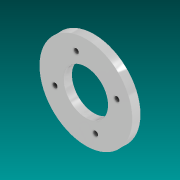
# Autodesk Inventor part: lagerblokje
Saved by Autodesk Inventor 2020.3 (Build 243373000, 373)
## iProperties
Created: 2020-05-22
Part Number: lagerblokje
Material: Aluminum 6061
Document SubType Name: Modeling
Designer: Svend
Density: 2.7 g/cm^3
Appearance: Aluminum - Polished
Author: Svend
Autodesk Inventor part; units mm, degrees
ref_plane "YZ Plane" through (0, 0, 0) normal (1, 0, 0) x (0, 1, 0)
ref_plane "XZ Plane" through (0, 0, 0) normal (0, 1, 0) x (-1, 0, 0)
ref_plane "XY Plane" through (0, 0, 0) normal (0, 0, 1) x (1, 0, 0)
ref_plane "Work Plane1" through (0, 0, 0) normal (0, 0, 1) x (1, 0, 0)
ref_plane "Work Plane2" through (0, 0, 0) normal (0, 0, 1) x (1, 0, 0)
sketch "Sketch2" plane through (0, 0, 0) normal (0, 0, 1) x (1, 0, 0)
  circle A0 centre (-137.1735, 0) radius 1.55
  circle A1 centre (-165.1735, -28) radius 1.55
  circle A2 centre (-165.1735, 28) radius 1.55
  circle A3 centre (-184.9724, -19.799) radius 1.55
  circle A4 centre (-145.3745, 19.799) radius 1.55
  circle A5 centre (-145.3745, -19.799) radius 1.55
  circle A6 centre (-184.9724, 19.799) radius 1.55
  circle A7 centre (-193.1735, 0) radius 1.55
  circle A8 centre (-165.1735, 0) radius 32.5
  circle A9 centre (-165.1735, 0) radius 22.8355
  circle A10 centre (-165.1735, 0) radius 11
  arc A11 (-152.3597, 3.5298) -> (-152.6156, 4.3532) centre (-149.894, 4.7473) ccw
  arc A12 (-152.6156, 4.3532) -> (-168.7032, 12.8137) centre (-165.1735, 0) ccw
  arc A13 (-168.7032, 12.8137) -> (-169.5266, 12.5579) centre (-169.9208, 15.2795) ccw
  arc A14 (-169.5266, 12.5579) -> (-177.9872, -3.5298) centre (-165.1735, 0) ccw
  arc A15 (-177.9872, -3.5298) -> (-177.7313, -4.3532) centre (-180.4529, -4.7473) ccw
  arc A16 (-177.7313, -4.3532) -> (-161.6437, -12.8137) centre (-165.1735, 0) ccw
  arc A17 (-161.6437, -12.8137) -> (-160.8203, -12.5579) centre (-160.4261, -15.2795) ccw
  arc A18 (-160.8203, -12.5579) -> (-152.3597, 3.5298) centre (-165.1735, 0) ccw
  circle A19 centre (-165.1735, 0) radius 20.2623
  circle A20 centre (-169.9208, 15.2795) radius 1.55
  circle A21 centre (-160.4261, -15.2795) radius 1.55
  circle A22 centre (-180.4529, -4.7473) radius 1.55
  circle A23 centre (-149.894, 4.7473) radius 1.55
  circle A24 centre (-165.1735, 0) radius 13.291
  point P0 (0, 0)
extrude "Extrusion2" add sketch "Sketch2" along normal blind 4 contours A9 | A24 A11 | A18 A24 A16 A14 A12 | A24 A13 | A17 A24 | A24 A15 | A19 | A20 | A21 | A22 | A23
sketch "Sketch3" plane through (-165.1735, 0, 0) normal (0, 0, -1) x (-1, 0, 0)
  point P0 (-165.1735, 0)
  point P1 (-15.2795, 4.7473)
  point P2 (4.7473, 15.2795)
  point P3 (15.2795, -4.7473)
  point P4 (-4.7473, -15.2795)
hole "Hole1" at (-149.894, 4.7473, 0) at (-169.9208, 15.2795, 0) at (-180.4529, -4.7473, 0) at (-160.4261, -15.2795, 0) direction (0, 0, 1) diameter 2.459 end through all thread size "M3x0.5" class "6H" standard "ISO Metric profile"
body "Solid2"
